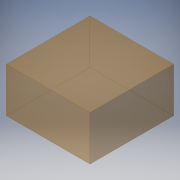
# Autodesk Inventor part: maxVolumeForLowBot
Saved by Autodesk Inventor 2016 SP1 (Build 200210100, 210)
## iProperties
Created: 2016-01-12
Part Number: maxVolumeForLowBot
Material: Polycarbonate, Smoke
Document SubType Name: Modeling
Designer: steele
Density: 1.2 g/cm^3
Appearance: Polycarbonate - Smoked
Author: steele
Autodesk Inventor part; units mm, degrees
ref_plane "YZ Plane" through (0, 0, 0) normal (1, 0, 0) x (0, 1, 0)
ref_plane "XZ Plane" through (0, 0, 0) normal (0, 1, 0) x (-1, 0, 0)
ref_plane "XY Plane" through (0, 0, 0) normal (0, 0, 1) x (1, 0, 0)
sketch "Sketch2" plane through (0, 0, 0) normal (0, 1, 0) x (-1, 0, 0)
  line L0 (381, 381) -> (-381, 381)
  line L1 (-381, 381) -> (-381, -381)
  line L2 (-381, -381) -> (381, -381)
  line L3 (381, -381) -> (381, 381)
  line L4 (381, 381) -> (-381, -381) construction
  line L5 (-381, 381) -> (381, -381) construction
  point P0 (0, 0)
  dimension "d4" = 762
  dimension "d5" = 762
  constraints: 12 end point, 2 midpoint, 2 parallel, 1 horizontal, 1 perpendicular
  measures "d4" distance of L0.start L0.end
  measures "d5" distance of L2.end L0.start
extrude "Extrusion1" add sketch "Sketch2" along normal blind 406.4
equation "\"d4\" = width"
equation "\"d5\" = length"
equation "\"width\" = 762"
equation "\"length\" = 762"
equation "\"height\" = 406.4"
equation "\"perimeter\" = 2 * width + 2 * length"
body "Solid1"
